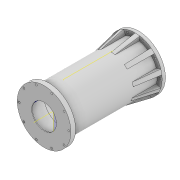
# Autodesk Inventor part: Anglerfish_Tube_v0
Saved by Autodesk Inventor 2022 (Build 260153000, 153)
## iProperties
Created: 2022-04-02
Part Number: Anglerfish_Tube_v0
Material: Generic
Document SubType Name: Modeling
Designer: Prakash Lab
Density: 1 g/cm^3
Appearance: Default
Author: Prakash Lab
Autodesk Inventor part; units mm, degrees
ref_plane "YZ Plane" through (0, 0, 0) normal (1, 0, 0) x (0, 1, 0)
ref_plane "Work Plane1" through (31.9356, -63.7595, -125.1157) normal (0, 0, -1) x (0, 1, 0)
sketch "Sketch1" plane through (0, 0, 0) normal (0, 0, 1) x (1, 0, 0)
  arc A0 (25.583, -14.3828) -> (8.2589, -31.7069) centre (33.1356, -39.2595) ccw projected
  circle A1 centre (33.1356, -39.2595) radius 33
  circle A2 centre (33.1356, -39.2595) radius 28
  point P0 (0, 0)
  dimension "d0" = 66
  dimension "d1" = 5
  constraints: 2 centre point, 1 coincident
  measures "d0" diameter of A1
  measures "d1" radial gap between concentric circles of A1 A2
extrude "Extrusion1" add sketch "Sketch1" against normal blind 135
sketch "Sketch2" plane through (33.1356, -39.2595, 0) normal (0, 0, 1) x (1, 0, 0)
  circle A0 centre (0, 0) radius 33 projected
  circle A1 centre (0, 0) radius 28 projected
  circle A2 centre (0, 0) radius 18.5
  circle A3 centre (0, 0) radius 40
  point P0 (-33.1356, 39.2595)
  dimension "d4" = 37
  dimension "d5" = 80
  constraints: 2 centre point, 2 coincident
  measures "d4" diameter of A2
  measures "d5" diameter of A3
extrude "Extrusion2" add sketch "Sketch2" along normal blind 1 contours A0 | A1 | A3
sketch "Sketch3" plane through (33.1356, -39.2595, 1) normal (0, 0, 1) x (1, 0, 0)
  circle A0 centre (0, 0) radius 40 projected
  circle A1 centre (0, 0) radius 18.5 projected
  circle A2 centre (37, 0) radius 1.4
  point P0 (-33.1356, 39.2595)
  dimension "d8" = 2.8
  dimension "d9" = 37
  constraints: 1 centre point
  measures "d8" diameter of A2
  measures "d9" distance of A2.centre A0.centre
extrude "Extrusion3" cut sketch "Sketch3" against normal through all contours A2
pattern_circular "Circular Pattern1" count 10 over 360 about axis through (33.1356, -39.2595, 0) along (0, 0, 1) of "Extrusion3"
chamfer "Chamfer1" distance 2 angle 45 1 edges at (0.1356, -39.2595, 0)
ref_plane "Work Plane2" through (31.9356, -63.7595, -32.1157) normal (0, 0, 1) x (1, 0, 0)
sketch "Sketch5" plane through (33.1356, -39.2595, -135) normal (0, 0, -1) x (-1, 0, 0)
  arc A0 (-1.2, 30.5) -> (-7.2, 24.5) centre (-1.2, 24.5) ccw projected
  arc A1 (7.2, 24.5) -> (1.2, 30.5) centre (1.2, 24.5) ccw projected
  arc A2 (-7.2, -24.5) -> (-1.2, -30.5) centre (-1.2, -24.5) ccw projected
  arc A3 (1.2, -30.5) -> (7.2, -24.5) centre (1.2, -24.5) ccw projected
  line L0 (-1.2, -30.5) -> (1.2, -30.5) projected
  line L1 (7.2, -24.5) -> (7.2, 24.5) projected
  line L2 (-7.2, 24.5) -> (-7.2, -24.5) projected
  line L3 (1.2, 30.5) -> (-1.2, 30.5) projected
  arc A4 (-1.2, 30.8) -> (-7.5, 24.5) centre (-1.2, 24.5) ccw
  line L4 (-1.2, 30.8) -> (1.2, 30.8)
  arc A5 (7.5, 24.5) -> (1.2, 30.8) centre (1.2, 24.5) ccw
  line L5 (7.5, 24.5) -> (7.5, -24.5)
  arc A6 (1.2, -30.8) -> (7.5, -24.5) centre (1.2, -24.5) ccw
  line L6 (1.2, -30.8) -> (-1.2, -30.8)
  arc A7 (-7.5, -24.5) -> (-1.2, -30.8) centre (-1.2, -24.5) ccw
  line L7 (-7.5, -24.5) -> (-7.5, 24.5)
  point P0 (33.1356, 39.2595)
  dimension "d22" = 0.3
  constraints: 8 end point, 8 point on circle, 4 centre point, 7 other
  measures "d22" radial gap between concentric circles of A0 A4
extrude "Extrusion5" cut sketch "Sketch5" against normal up to surface (102.8843 mm away) contours L3 A1 L1 A3 L0 A2 L2 A0 | L4 A5 L5 A6 L6 A7 L7 A4
sketch "Sketch6" plane through (33.1356, -39.2595, -135) normal (0, 0, -1) x (-1, 0, 0)
  circle A0 centre (0, 0) radius 33 projected
  circle A1 centre (0, 0) radius 40 projected
  circle A2 centre (0, 0) radius 40 projected
  circle A3 centre (-37, 0) radius 1.4 projected
  circle A4 centre (-29.9336, 21.7481) radius 1.4 projected
  circle A5 centre (-11.4336, 35.1891) radius 1.4 projected
  circle A6 centre (11.4336, 35.1891) radius 1.4 projected
  circle A7 centre (29.9336, 21.7481) radius 1.4 projected
  circle A8 centre (37, 0) radius 1.4 projected
  circle A9 centre (29.9336, -21.7481) radius 1.4 projected
  circle A10 centre (11.4336, -35.1891) radius 1.4 projected
  circle A11 centre (-11.4336, -35.1891) radius 1.4 projected
  circle A12 centre (-29.9336, -21.7481) radius 1.4 projected
  circle A13 centre (0, 0) radius 35 projected
  arc A14 (6.9247, -27.1302) -> (6.9247, 27.1302) centre (0, 0) ccw projected
  arc A15 (-6.9247, 27.1302) -> (-6.9247, -27.1302) centre (0, 0) ccw projected
  arc A16 (-6.9247, -27.1302) -> (-1.2, -30.8) centre (-1.2, -24.5) ccw projected
  arc A17 (1.2, -30.8) -> (6.9247, -27.1302) centre (1.2, -24.5) ccw projected
  line L0 (1.2, -30.8) -> (-1.2, -30.8) projected
  arc A18 (6.9247, 27.1302) -> (1.2, 30.8) centre (1.2, 24.5) ccw projected
  line L1 (-1.2, 30.8) -> (1.2, 30.8) projected
  arc A19 (-1.2, 30.8) -> (-6.9247, 27.1302) centre (-1.2, 24.5) ccw projected
  point P0 (33.1356, 39.2595)
extrude "Extrusion6" add sketch "Sketch6" along normal blind 5 contours A0 | A1 | A13
ref_plane "Work Plane3" through (33.1356, -39.2595, -78.6157) normal (1, 0, 0) x (0, 0, -1)
sketch "Sketch7" plane through (33.1356, -39.2595, -78.6157) normal (1, 0, 0) x (0, 0, -1)
  line L0 (-76.6157, -33) -> (56.3843, -33) projected
  line L1 (56.3843, -40) -> (56.3843, 40) projected
  line L2 (56.3843, -40) -> (20.591, -33)
  line L3 (56.3843, -40) -> (56.3843, -33)
  line L4 (-106.6157, 0) -> (89.3843, 0) projected
  point P0 (-78.6157, 39.2595)
  constraints: 4 end point, 1 perpendicular, 1 point on line
revolve "Revolution1" add sketch "Sketch7" angle 10 about axis through (33.1356, -39.2595, 0) along (0, 0, -1)
pattern_circular "Circular Pattern2" count 10 over 360 about axis through (33.1356, -39.2595, 0) along (0, 0, -1) of "Revolution1"
sketch "Sketch8" plane through (33.1356, -39.2595, 0) normal (0, 0, -1) x (-1, 0, 0)
  circle A0 centre (0, 0) radius 40 projected
  circle A1 centre (-37, 0) radius 1.4 projected
  circle A2 centre (-29.9336, 21.7481) radius 1.4 projected
  circle A3 centre (-11.4336, 35.1891) radius 1.4 projected
  circle A4 centre (11.4336, 35.1891) radius 1.4 projected
  circle A5 centre (29.9336, 21.7481) radius 1.4 projected
  circle A6 centre (37, 0) radius 1.4 projected
  circle A7 centre (29.9336, -21.7481) radius 1.4 projected
  circle A8 centre (11.4336, -35.1891) radius 1.4 projected
  circle A9 centre (-11.4336, -35.1891) radius 1.4 projected
  circle A10 centre (-29.9336, -21.7481) radius 1.4 projected
  circle A11 centre (0, 0) radius 35 projected
  circle A12 centre (0, 0) radius 33 projected
  point P0 (33.1356, 39.2595)
extrude "Extrusion7" add sketch "Sketch8" along normal blind 6 contours A0 | A11
ref_plane "Work Plane4" through (33.1356, -57.7595, -25.1157) normal (-1, 0, 0) x (0, 1, 0)
sketch "Sketch9" plane through (33.1356, -57.7595, -25.1157) normal (-1, 0, 0) x (0, 1, 0)
  line L0 (-7.5, 2) -> (-7.5, -7.5)
  line L1 (-9.5, 7) -> (-9.5, -25.1157) projected
  line L2 (-9.5, 7) -> (-8, 0.0442)
  line L3 (-8, 0.0442) -> (-8, -15.215)
  line L4 (-8, -15.215) -> (-8, -25.1157)
  line L5 (46.5, -25.1157) -> (-9.5, -25.1157) projected
  line L6 (-8, -25.1157) -> (-9.5, -25.1157)
  line L7 (-9.5, -25.1157) -> (-9.5, 7)
  line L8 (18.5, -53.1157) -> (18.5, 142.8843) projected
  point P0 (57.7595, -25.1157)
  dimension "d33" = 0.5
  constraints: 12 end point, 2 perpendicular, 2 vertical, 1 point on line, 2 other
  measures "d33" distance between parallel lines of L0 L3
revolve "Revolution2" add sketch "Sketch9" angle 360 about axis through (33.1356, -39.2595, 0) along (0, 0, -1)
ref_plane "Work Plane5" through (31.9356, -39.2595, -119.1157) normal (0, 1, 0) x (0, 0, 1)
sketch "Sketch10" plane through (31.9356, -39.2595, -119.1157) normal (0, 1, 0) x (0, 0, 1)
  line L0 (92, 27.2) -> (111.5, 27.2)
  line L1 (92, -24.8) -> (111.5, -24.8)
  line L2 (-20.8843, 29.2) -> (87, 29.2) projected
  line L3 (-20.8843, -26.8) -> (87, -26.8) projected
  point P0 (119.1157, -31.9356)
  constraints: 4 end point, 2 horizontal, 4 other
body "Solid1"
